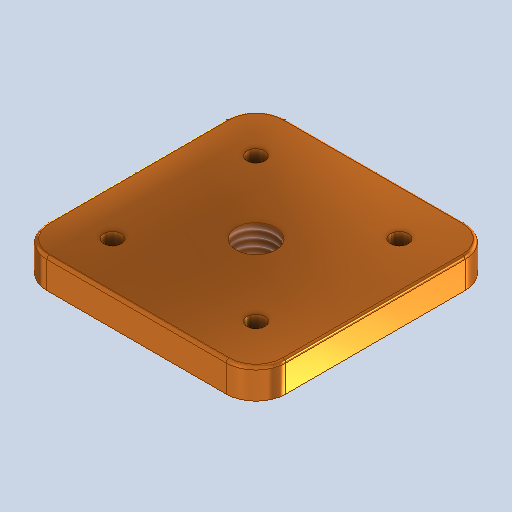
# Autodesk Inventor part: 27
Saved by Autodesk Inventor 2025.1 (Build 291241000, 241)
## iProperties
Created: 2024-09-17
Part Number: 27
Material: Gold
Document SubType Name: Modeling
Designer: ffogue
Density: 19.3 g/cm^3
Appearance: Metal 1600F Hot
Author: ffogue
Autodesk Inventor part; units mm, degrees
ref_plane "YZ Plane" through (0, 0, 0) normal (1, 0, 0) x (0, 1, 0)
ref_plane "XZ Plane" through (0, 0, 0) normal (0, 1, 0) x (-1, 0, 0)
ref_plane "XY Plane" through (0, 0, 0) normal (0, 0, 1) x (1, 0, 0)
sketch "Sketch1" plane through (0, 0, 0) normal (0, 0, 1) x (1, 0, 0)
  line L0 (-20, -20) -> (20, -20)
  line L1 (20, -20) -> (20, 20)
  line L2 (20, 20) -> (-20, 20)
  line L3 (-20, 20) -> (-20, -20)
  line L4 (-20, -20) -> (20, 20) construction
  line L5 (20, -20) -> (-20, 20) construction
  point P0 (0, 0)
  dimension "d0" = 40
  dimension "d1" = 40
  constraints: 12 end point, 2 midpoint, 2 parallel, 1 horizontal, 1 perpendicular
  measures "d0" distance of L1.end L2.end
  measures "d1" distance of L2.end L0.start
extrude "Extrusion1" add sketch "Sketch1" along normal blind 5
sketch "Sketch2" plane through (0, 0, 5) normal (0, 0, 1) x (1, 0, 0)
  point P0 (0, 0)
  point P1 (-12, 12)
  point P2 (12, 12)
  point P3 (12, -12)
  point P4 (-12, -12)
  point P5 (0, 0)
  dimension "d4" = 24
  dimension "d5" = 12
  dimension "d6" = 24
  dimension "d7" = 12
  constraints: 2 horizontal alignment, 2 vertical alignment, 1 coincident
  measures "d4" distance of point (12, 12) point (-12, 12)
  measures "d5" horizontal distance of point (0, 0) point (-12, 12)
  measures "d6" distance of point (-12, -12) point (-12, 12)
  measures "d7" horizontal distance of point (0, 0) point (-12, -12)
hole "Hole1" at (-12, 12, 5) at (12, 12, 5) at (12, -12, 5) at (-12, -12, 5) direction (0, 0, -1) diameter 3 depth 5
hole "Hole2" at (0, 0, 5) direction (0, 0, -1) diameter 6.647 depth 5 thread size "M8x1.25" class "6H" standard "ISO Metric profile"
fillet "Fillet1" radius 5 4 edges at (20, 20, 2.5) (20, -20, 2.5) (-20, -20, 2.5) (-20, 20, 2.5)
fillet "Fillet2" radius 0.5 8 edges at (18.5355, -18.5355, 5) (20, 0, 5) (18.5355, 18.5355, 5) (0, 20, 5) (-18.5355, 18.5355, 5) (-20, 0, 5) (-18.5355, -18.5355, 5) (0, -20, 5)
equation "\"d5\" = 0.5 * d4"
equation "\"d7\" = 0.5 * d6"
body "Solid1"
